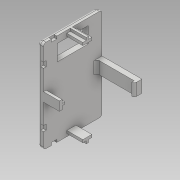
# Autodesk Inventor part: door
Saved by Autodesk Inventor 2018.2 (Build 222227000, 227)
## iProperties
Created: 2019-05-29
Part Number: door
Material: Generico
Document SubType Name: Modeling
Designer: fabio
Density: 1 g/cm^3
Appearance: Default
Author: fabio
Autodesk Inventor part; units mm, degrees
ref_plane "YZ Plane" through (0, 0, 0) normal (1, 0, 0) x (0, 1, 0)
ref_plane "XZ Plane" through (0, 0, 0) normal (0, 1, 0) x (-1, 0, 0)
ref_plane "XY Plane" through (0, 0, 0) normal (0, 0, 1) x (1, 0, 0)
sketch "Schizzo1" plane through (0, 0, 0) normal (1, 0, 0) x (0, 1, 0)
  line L0 (-11, 17.3) -> (11, 17.3)
  line L1 (11, 17.3) -> (11, -17.3)
  line L2 (11, -17.3) -> (-11, -17.3)
  line L3 (-11, -17.3) -> (-11, 17.3)
  line L4 (-11, 17.3) -> (11, -17.3) construction
  line L5 (11, 17.3) -> (-11, -17.3) construction
  point P0 (0, 0)
  dimension "d0" = 34.6
  dimension "d1" = 22
  constraints: 12 end point, 2 midpoint, 2 parallel, 1 horizontal, 1 perpendicular
  measures "d0" distance of L2.end L0.start
  measures "d1" distance of L1.end L2.end
extrude "Estrusione1" add sketch "Schizzo1" along normal blind 2
sketch "Schizzo8" plane through (2, 0, 0) normal (1, 0, 0) x (0, 0, -1)
  line L0 (-15.3, 8) -> (15.3, 8)
  line L1 (15.3, 8) -> (15.3, -9)
  line L2 (15.3, -9) -> (-15.3, -9)
  line L3 (-15.3, -9) -> (-15.3, 8)
  line L4 (-17.3, 11) -> (-17.3, -11) projected
  line L5 (-17.3, -11) -> (17.3, -11) projected
  line L6 (17.3, -11) -> (17.3, 11) projected
  line L7 (17.3, 11) -> (-17.3, 11) projected
  line L8 (-0.4, -9) -> (0.4, -9)
  line L9 (0.4, -9) -> (0.4, -10)
  line L10 (0.4, -10) -> (1.7, -10)
  line L11 (1.7, -10) -> (1.7, -11)
  line L12 (1.7, -11) -> (-1.7, -11)
  line L13 (-1.7, -11) -> (-1.7, -10)
  line L14 (-1.7, -10) -> (-0.4, -10)
  line L15 (-0.4, -10) -> (-0.4, -9)
  line L16 (-15.3, -2.2) -> (-16.3, -2.2)
  line L17 (-16.3, -2.2) -> (-16.3, -0.9)
  line L18 (-16.3, -0.9) -> (-17.3, -0.9)
  line L19 (-17.3, -0.9) -> (-17.3, -0.1)
  line L20 (-17.3, -0.1) -> (-16.3, -0.1)
  line L21 (-16.3, -0.1) -> (-16.3, 1.2)
  line L22 (-16.3, 1.2) -> (-15.3, 1.2)
  line L23 (-15.3, 1.2) -> (-15.3, -2.2)
  line L24 (0, 0) -> (0, 8)
  line L25 (15.3, -2.2) -> (16.3, -2.2)
  line L26 (16.3, -2.2) -> (16.3, -0.9)
  line L27 (16.3, -0.9) -> (17.3, -0.9)
  line L28 (17.3, -0.9) -> (17.3, -0.1)
  line L29 (17.3, -0.1) -> (16.3, -0.1)
  line L30 (16.3, -0.1) -> (16.3, 1.2)
  line L31 (16.3, 1.2) -> (15.3, 1.2)
  line L32 (15.3, 1.2) -> (15.3, -2.2)
  point P0 (0, -11)
  point P1 (-15.3, -0.5)
  dimension "d47" = 17
  dimension "d48" = 30.6
  dimension "d49" = 2
  dimension "d50" = 2
  dimension "d51" = 0.8
  dimension "d52" = 1.3
  dimension "d53" = 1.3
  dimension "d54" = 1
  dimension "d55" = 1
  dimension "d61" = 1
  dimension "d62" = 1
  dimension "d63" = 1
  dimension "d64" = 0.8
  dimension "d65" = 1.3
  dimension "d66" = 1.3
  constraints: 58 end point, 14 perpendicular, 8 symmetric about line, 5 midpoint, 4 horizontal, 2 parallel, 2 point on line
  measures "d47" distance of L0.end L1.end
  measures "d48" distance of L1.end L2.end
  measures "d49" distance between parallel lines of L6 L1
  measures "d50" distance between parallel lines of L5 L2
  measures "d51" distance of L8.start L8.end
  measures "d52" distance of L13.end L14.end
  measures "d53" distance of L9.end L10.end
  measures "d54" distance of L8.end L9.end
  measures "d55" distance of L10.end L11.end
  measures "d61" distance of L16.start L16.end
  measures "d62" distance of L21.end L22.end
  measures "d63" distance of L17.end L18.end
  measures "d64" distance of L18.end L19.end
  measures "d65" distance of L20.end L21.end
  measures "d66" distance of L16.end L17.end
extrude "Estrusione9" add sketch "Schizzo8" along normal blind 6 contours L3 L16 L17 L18 L4 L20 L21 L22 | L31 L30 L29 L6 L27 L26 L25 L1 | L2 L9 L10 L11 L5 L13 L14 L15
sketch "Schizzo4" plane through (2, 0, 0) normal (1, 0, 0) x (0, 0, -1)
  line L0 (17.3, 11) -> (-17.3, 11) projected
  line L1 (-2.3, 11) -> (2.3, 11)
  line L2 (2.3, 11) -> (2.3, 9)
  line L3 (2.3, 9) -> (-2.3, 9)
  line L4 (-2.3, 9) -> (-2.3, 11)
  point P0 (0, 0)
  point P1 (0, 11)
  dimension "d19" = 2
  dimension "d20" = 4.6
  constraints: 8 end point, 2 midpoint, 2 parallel, 1 horizontal, 1 perpendicular
  measures "d19" distance of L1.end L2.end
  measures "d20" distance of L2.end L3.end
extrude "Estrusione4" add sketch "Schizzo4" along normal blind 15
sketch "Schizzo5" plane through (2, 9, 2.3) normal (0, 0, 1) x (1, 0, 0)
  line L0 (0, 0) -> (15, 0) projected
  line L1 (0, 0) -> (15, 0) projected
  line L2 (14.1, 0) -> (14.1, -0.9)
  arc A0 (14.1, -0.9) -> (15, 0) centre (14.1, 0) ccw
  point P0 (-2, -9)
  dimension "d23" = 0.9
  constraints: 2 end point, 2 point on circle, 1 centre point, 1 coincident, 1 perpendicular, 1 point on line
  measures "d23" distance of L2.start L2.end
extrude "Estrusione5" add sketch "Schizzo5" against normal up to surface (4.6 mm away)
sketch "Schizzo6" plane through (2, 0, 0) normal (-1, 0, 0) x (0, 0, 1)
  line L0 (-17.3, -11) -> (17.3, -11) projected
  line L1 (17.3, -11) -> (17.3, 11) projected
  line L2 (-11.3, -10) -> (-9.3, -10)
  line L3 (-9.3, -10) -> (-9.3, -11)
  line L4 (-9.3, -11) -> (-11.3, -11)
  line L5 (-11.3, -11) -> (-11.3, -10)
  line L6 (0, 0) -> (0, -11)
  line L7 (-17.3, -6) -> (-16.3, -6)
  line L8 (-16.3, -6) -> (-16.3, -8)
  line L9 (-16.3, -8) -> (-17.3, -8)
  line L10 (-17.3, -8) -> (-17.3, -6)
  line L11 (11.3, -10) -> (9.3, -10)
  line L12 (9.3, -10) -> (9.3, -11)
  line L13 (9.3, -11) -> (11.3, -11)
  line L14 (11.3, -11) -> (11.3, -10)
  line L15 (17.3, -6) -> (16.3, -6)
  line L16 (16.3, -6) -> (16.3, -8)
  line L17 (16.3, -8) -> (17.3, -8)
  line L18 (17.3, -8) -> (17.3, -6)
  line L19 (-17.3, 11) -> (-17.3, -11) projected
  dimension "d26" = 2
  dimension "d27" = 1
  dimension "d29" = 1
  dimension "d32" = 3
  dimension "d33" = 6
  dimension "d36" = 2
  constraints: 34 end point, 8 symmetric about line, 4 parallel, 2 collinear, 2 horizontal, 2 perpendicular, 1 midpoint
  measures "d26" distance of L3.end L4.end
  measures "d27" distance of L4.end L2.start
  measures "d29" distance of L8.end L9.end
  measures "d32" distance between parallel lines of L0 L9
  measures "d33" distance between parallel lines of L19 L5
  measures "d36" distance of L7.end L8.end
extrude "Estrusione7" cut sketch "Schizzo6" along normal blind 1
sketch "Schizzo7" plane through (0, 0, 0) normal (-1, 0, 0) x (0, 0, 1)
  line L0 (8.8, 5.75) -> (14.8, 5.75)
  line L1 (14.8, 5.75) -> (14.8, -5.75)
  line L2 (14.8, -5.75) -> (8.8, -5.75)
  line L3 (8.8, -5.75) -> (8.8, 5.75)
  line L4 (17.3, -11) -> (17.3, 11) projected
  line L5 (17.3, 11) -> (-17.3, 11) projected
  line L6 (-17.3, 11) -> (-17.3, -11) projected
  line L7 (-17.3, -11) -> (17.3, -11) projected
  line L8 (-17.3, 0) -> (17.3, 0)
  point P0 (0, 0)
  point P1 (14.8, 0)
  dimension "d39" = 6
  dimension "d40" = 11.5
  dimension "d42" = 2.5
  constraints: 10 end point, 3 midpoint, 2 parallel, 1 horizontal, 1 perpendicular, 1 point on line
  measures "d39" distance of L1.end L2.end
  measures "d40" distance of L0.end L1.end
  measures "d42" distance between parallel lines of L4 L1
extrude "Estrusione8" cut sketch "Schizzo7" against normal up to surface (2 mm away) contours L0 L1 L8 L3 | L8 L1 L2 L3
fillet "Raccordo1" radius 1 8 edges at (0, 11, 0) (0, 0, -17.3) (0, -11, 0) (0, 0, 17.3) (1, -11, 17.3) (1, -11, -17.3) (1, 11, -17.3) (1, 11, 17.3)
fillet "Raccordo2" radius 1 1 edges at (2, 9, 0)
equation "\"d53\" = d52"
equation "\"d61\" = d54"
equation "\"d62\" = d61"
equation "\"d63\" = d61"
equation "\"d66\" = d65"
equation "\"d36\" = d26"
